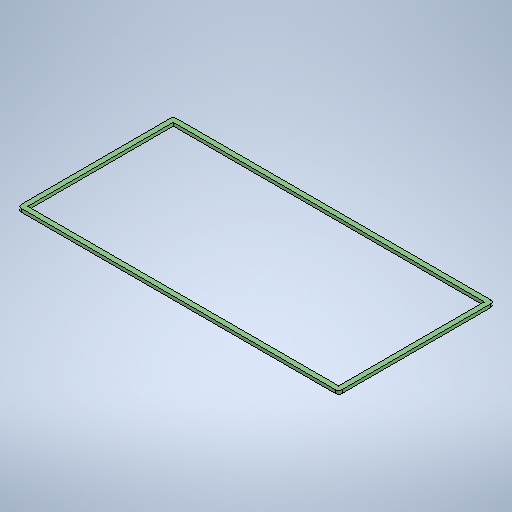
# Autodesk Inventor part: PinecilCaseBorder
Saved by Autodesk Inventor 2026 (Build 300175050, 175E)
## iProperties
Created: 2025-10-10
Part Number: PinecilCaseBorder
Material: ABS Plastic
Document SubType Name: Modeling
Designer: Nicholas M
Density: 1.06 g/cm^3
Appearance: Smooth - Dark Forest Green
Author: Nicholas M
Autodesk Inventor part; units mm, degrees
ref_plane "YZ Plane" through (0, 0, 0) normal (1, 0, 0) x (0, 1, 0)
ref_plane "XZ Plane" through (0, 0, 0) normal (0, 1, 0) x (-1, 0, 0)
ref_plane "XY Plane" through (0, 0, 0) normal (0, 0, 1) x (1, 0, 0)
sketch "Sketch1" plane through (0, 0, 0) normal (0, 1, 0) x (-1, 0, 0)
  line L0 (1.27, 0) -> (121.92, 0)
  line L1 (123.19, -1.27) -> (123.19, -58.42)
  line L2 (121.92, -59.69) -> (1.27, -59.69)
  line L3 (0, -58.42) -> (0, -1.27)
  arc A0 (123.19, -1.27) -> (121.92, 0) centre (121.92, -1.27) ccw
  arc A1 (121.92, -59.69) -> (123.19, -58.42) centre (121.92, -58.42) ccw
  arc A2 (0, -58.42) -> (1.27, -59.69) centre (1.27, -58.42) ccw
  arc A3 (1.27, 0) -> (0, -1.27) centre (1.27, -1.27) ccw
  line L4 (121.285, -1.905) -> (1.905, -1.905)
  line L5 (1.905, -1.905) -> (1.905, -57.785)
  line L6 (1.905, -57.785) -> (121.285, -57.785)
  line L7 (121.285, -57.785) -> (121.285, -1.905)
  point P0 (0, 0)
  point P1 (123.19, -59.69)
  point P2 (123.19, 0)
  point P3 (0, -59.69)
  dimension "d0" = 59.69
  dimension "d1" = 123.19
  dimension "d2" = 1.27
  dimension "d3" = 1.27
  dimension "d4" = 1.905
  constraints: 16 end point, 8 point on circle, 8 point on line, 8 tangent, 4 centre point, 4 parallel, 2 equal radius, 2 perpendicular, 1 horizontal, 3 other
  measures "d0" distance of point (123.19, 0) point (123.19, -59.69)
  measures "d1" distance of point (123.19, -59.69) point (0, -59.69)
  measures "d2" radius of A0
  measures "d3" radius of A3
  measures "d4" distance between parallel lines of L0 L4
extrude "Extrusion1" add sketch "Sketch1" along normal blind 1.27
equation "\"d3\" = d2"
body "Solid1"
